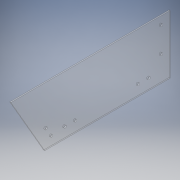
# Autodesk Inventor part: PaddleCollection2.1Casing
Saved by Autodesk Inventor 2019 (Build 230136000, 136)
## iProperties
Created: 2018-10-20
Part Number: PaddleCollection2.1Casing
Material: Polycarbonate, Clear
Document SubType Name: Modeling
Designer: User
Density: 1.2 g/cm^3
Appearance: Polycarbonate - Clear
Mass: 36.0285 g
Surface Area: 334.77 cm^2
Volume: 30.0237 cm^3
Author: User
Autodesk Inventor part; units mm, degrees
ref_plane "YZ Plane" through (0, 0, 0) normal (1, 0, 0) x (0, 1, 0)
ref_plane "XZ Plane" through (0, 0, 0) normal (0, 1, 0) x (-1, 0, 0)
ref_plane "XY Plane" through (0, 0, 0) normal (0, 0, 1) x (1, 0, 0)
sketch "Sketch1" plane through (0, 0, 0) normal (1, 0, 0) x (0, 1, 0)
  line L0 (0, 0) -> (88.9, 0)
  line L1 (88.9, 0) -> (88.9, -241.8264)
  line L2 (88.9, -241.8264) -> (0, -241.8264)
  line L3 (0, -241.8264) -> (0, 0)
  line L4 (88.9, 0) -> (0, -51.3264)
  line L5 (88.9, 0) -> (191.5529, 0) construction
  dimension "d0" = 88.9
  dimension "d2" = 150
  dimension "d5" = 190.5
  constraints: 12 end point, 2 horizontal, 2 parallel, 1 equal length, 1 perpendicular, 1 point on line
  measures "d0" distance of L1.end L2.end
  measures "d2" angle of L4 L5
  measures "d5" distance from line of L2 L4.end
extrude "Extrusion1" add sketch "Sketch1" along normal blind 1.8542 contours L1 L2 L3 L4
sketch "Sketch2" plane through (1.8542, 0, 0) normal (1, 0, 0) x (0, 0, -1)
  line L0 (241.8264, 0) -> (241.8264, 88.9) projected
  line L1 (51.3264, 0) -> (241.8264, 0) projected
  line L2 (0, 88.9) -> (51.3264, 0) projected
  point P0 (0, 0)
  point P1 (82.2382, 16.002)
  point P2 (98.2382, 16.002)
  point P3 (193.5664, 16.002)
  point P4 (209.5664, 16.002)
  point P5 (53.6378, 28.0005)
  point P6 (61.7404, 13.9664)
  dimension "d6" = 16
  dimension "d8" = 16
  dimension "d9" = 16.002
  dimension "d10" = 16.002
  dimension "d11" = 16.002
  dimension "d12" = 16.002
  dimension "d13" = 159.5882
  dimension "d14" = 48.26
  dimension "d22" = 16.002
  dimension "d23" = 16.002
  dimension "d24" = 188.1886
  dimension "d25" = 180.086
  measures "d6" distance of point (98.238, 16.002) point (82.238, 16.002)
  measures "d8" distance of point (193.566, 16.002) point (209.566, 16.002)
  measures "d9" distance from line of L1 point (193.566, 16.002)
  measures "d10" distance from line of L1 point (209.566, 16.002)
  measures "d11" distance from line of L1 point (98.238, 16.002)
  measures "d12" distance from line of L1 point (82.238, 16.002)
  measures "d13" distance from line of point (82.238, 16.002) L0
  measures "d14" distance from line of point (193.566, 16.002) L0
  measures "d22" distance from line of L2 point (53.638, 28.001)
  measures "d23" distance from line of L2 point (61.74, 13.966)
  measures "d24" distance from line of L0 point (53.638, 28.001)
  measures "d25" distance from line of L0 point (61.74, 13.966)
hole "Hole1" at (1.8542, 16.002, -82.2382) at (1.8542, 16.002, -98.2382) at (1.8542, 16.002, -193.5664) at (1.8542, 16.002, -209.5664) at (1.8542, 28.0005, -53.6378) at (1.8542, 13.9664, -61.7404) direction (-1, 0, 0) diameter 3.81 depth 10.9728 tip angle 118
sketch "Sketch3" plane through (1.8542, 0, 0) normal (1, 0, 0) x (0, 0, -1)
  line L0 (241.8264, 0) -> (241.8264, 88.9) projected
  line L1 (51.3264, 0) -> (241.8264, 0) projected
  point P0 (0, 0)
  point P1 (228.5676, 76.2)
  point P2 (228.5676, 38.1)
  dimension "d26" = 13.2588
  dimension "d27" = 13.2588
  dimension "d28" = 76.2
  dimension "d29" = 38.1
  measures "d26" distance from line of point (228.568, 76.2) L0
  measures "d27" distance from line of L0 point (228.568, 38.1)
  measures "d28" distance from line of L1 point (228.568, 76.2)
  measures "d29" distance from line of L1 point (228.568, 38.1)
hole "Hole2" at (1.8542, 76.2, -228.5676) at (1.8542, 38.1, -228.5676) direction (-1, 0, 0) diameter 3.81 depth 10.9728 tip angle 118
equation "\"d8\" = d6"
equation "\"d10\" = d9"
equation "\"d11\" = d9"
equation "\"d12\" = d9"
equation "\"d22\" = d11"
equation "\"d23\" = d22"
equation "\"d27\" = d26"
body "Solid1"
